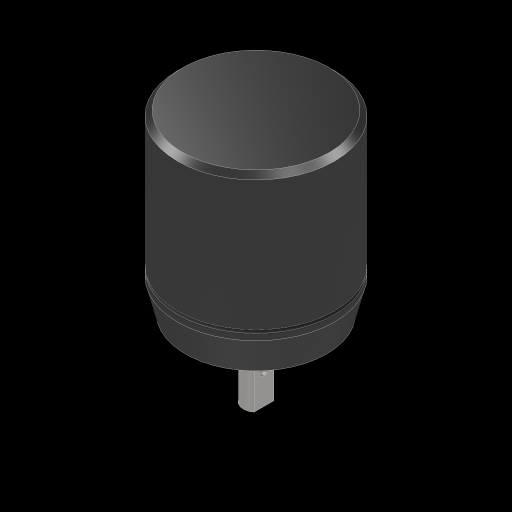
# Autodesk Inventor part: 5065
Saved by Autodesk Inventor 2023 (Build 270158030, 158C)
## iProperties
Created: 2022-10-21
Part Number: 5065
Material: Generic
Document SubType Name: Modeling
Designer: kumpu
Density: 4.593 g/cm^3
Appearance: Glossy - Black
Mass: 476.272 g
Surface Area: 164.006 cm^2
Volume: 103.695 cm^3
Author: kumpu
Autodesk Inventor part; units mm, degrees
ref_plane "YZ Plane" through (0, 0, 0) normal (1, 0, 0) x (0, 1, 0)
ref_plane "XZ Plane" through (0, 0, 0) normal (0, 1, 0) x (-1, 0, 0)
ref_plane "XY Plane" through (0, 0, 0) normal (0, 0, 1) x (1, 0, 0)
sketch "Sketch1" plane through (0, 0, 0) normal (0, 0, 1) x (1, 0, 0)
  line L0 (0, 55.5) -> (0, -24.2)
  line L1 (0, -24.2) -> (4, -24.2)
  line L2 (4, -24.2) -> (4, 0)
  line L3 (4, 0) -> (24.75, 0)
  line L4 (24.75, 0) -> (24.75, 55.5)
  line L5 (24.75, 55.5) -> (0, 55.5)
  line L6 (24.75, 12) -> (4, 12)
  line L7 (4, 12) -> (4, 13)
  line L8 (4, 13) -> (24.75, 13)
  line L9 (24.75, 13) -> (24.75, 12)
  point P0 (0, 0)
  point P1 (24.75, 13)
  dimension "d0" = 8
  dimension "d1" = 24.2
  dimension "d2" = 55.5
  dimension "d3" = 49.5
  dimension "d24" = 12
  dimension "d25" = 1
  constraints: 21 end point, 6 perpendicular, 3 point on line, 2 parallel, 1 collinear, 1 horizontal, 1 vertical
  measures "d0" diameter of L2 L0
  measures "d1" distance of L1.end L2.end
  measures "d2" distance of L3.end L4.end
  measures "d3" diameter of L4 L0
  measures "d24" distance between parallel lines of L3 L6
  measures "d25" distance of L6.end L7.end
revolve "Revolution1" add sketch "Sketch1" angle 360 about axis through (0, 55.5, 0) along (0, -1, 0) contours L5 L4 L8 L7 L6 L3 L2 L1 L0
sketch "Sketch2" plane through (0, 0, 0) normal (0, -1, 0) x (1, 0, 0)
  circle A0 centre (19, 0) radius 2
  circle A1 centre (0, 0) radius 4 construction
  line L0 (0, 0) -> (19, 0) construction
  circle A2 centre (0, 19) radius 2
  circle A3 centre (-19, 0) radius 2
  circle A4 centre (0, -19) radius 2
  point P0 (0, 0)
  dimension "d5" = 4
  dimension "d6" = 19
  dimension "d9" = 360
  constraints: 4 centre point, 2 end point, 1 horizontal, 9 other
  measures "d5" diameter of A0
  measures "d6" distance of L0.start L0.end
extrude "Extrusion1" cut sketch "Sketch2" against normal blind 5
sketch "Sketch3" plane through (0, -24.2, 0) normal (0, -1, 0) x (1, 0, 0)
  line L0 (2.5, 3.1225) -> (2.5, -3.1225)
  arc A0 (2.5, -3.1225) -> (2.5, 3.1225) centre (0, 0) ccw
  circle A1 centre (0, 0) radius 4 construction
  point P0 (0, 0)
  dimension "d13" = 2.5
  constraints: 2 concentric, 2 end point, 2 point on circle, 1 centre point, 1 vertical
  measures "d13" distance from line of A0.centre L0
extrude "Extrusion2" cut sketch "Sketch3" against normal blind 18
sketch "Sketch4" plane through (2.5, -24.2, 3.1225) normal (1, 0, 0) x (0, 0, -1)
  line L0 (-0.8775, 0) -> (7.1225, 0) construction
  line L1 (3.1225, 0) -> (3.1225, 10) construction
  point P0 (3.1225, 24.2)
  point P1 (0, 0)
  point P2 (6.245, 0)
  dimension "d16" = 10
  constraints: 2 end point, 1 coincident, 1 midpoint, 1 vertical
  measures "d16" distance of L1.start L1.end
hole "Hole1" at (2.5, -14.2, 0) direction (-1, 0, 0) diameter 3.2 depth 1 tip angle 118
chamfer "Chamfer1" distance 1.6 angle 45 1 edges at (-24.75, 55.5, 0)
chamfer "Chamfer2" distance 2.5 distance2 10 1 edges at (-24.75, 0, 0) measured on face at (-24.25, 0, 0)
body "Solid1"
